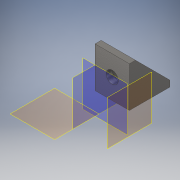
# Autodesk Inventor part: Corner Piece
Saved by Autodesk Inventor 2017 (Build 210142000, 142)
## iProperties
Part Number: Corner Piece
Material: Aluminum 6061-AHC
Document SubType Name: Modeling
Designer: Till
Density: 2.7 g/cm^3
Appearance: Galvanisiert
Author: Till
Autodesk Inventor part; units mm, degrees
ref_plane "YZ Plane" through (0, 0, 0) normal (1, 0, 0) x (0, 1, 0)
ref_plane "XZ Plane" through (0, 0, 0) normal (0, 1, 0) x (-1, 0, 0)
ref_plane "XY Plane" through (0, 0, 0) normal (0, 0, 1) x (1, 0, 0)
ref_plane "Arbeitsebene7" through (0, 0, 0) normal (0, 0, 1) x (1, 0, 0)
sketch "Skizze1" plane through (0, 0, 0) normal (0, 0, 1) x (1, 0, 0)
  line L0 (12, 20) -> (17, 20) projected
  line L1 (0, 20) -> (5, 20) projected
  line L2 (17, 20) -> (0, 20)
  line L3 (0, 20) -> (0, 40)
  line L4 (0, 40) -> (17, 40)
  line L5 (17, 40) -> (17, 20)
  point P0 (0, 0)
  dimension "d0" = 20
  constraints: 8 end point, 3 perpendicular, 1 collinear
  measures "d0" distance of L1.start L3.end
extrude "Extrusion1" add sketch "Skizze1" along normal blind 3
ref_plane "Arbeitsebene6" through (5, 20, 0) normal (0, 1, 0) x (-1, 0, 0)
sketch "Skizze2" plane through (5, 20, 0) normal (0, 1, 0) x (-1, 0, 0)
  line L0 (-12, 0) -> (-12, 400) projected
  line L1 (5, 3) -> (-12, 3) projected
  line L2 (-12, 3) -> (5, 3)
  line L3 (5, 3) -> (5, 20)
  line L4 (5, 20) -> (-12, 20)
  line L5 (-12, 20) -> (-12, 3)
  point P0 (5, 0)
  dimension "d3" = 17
  constraints: 8 end point, 2 parallel, 1 horizontal, 1 perpendicular
  measures "d3" distance of L3.end L2.end
extrude "Extrusion2" add sketch "Skizze2" along normal blind 3
ref_plane "Arbeitsebene5" through (0, 20, 0) normal (-1, 0, 0) x (0, 0, 1)
sketch "Skizze4" plane through (0, 20, 0) normal (-1, 0, 0) x (0, 0, 1)
  line L0 (3, 3) -> (3, 20) projected
  line L1 (20, 3) -> (3, 3) projected
  line L2 (3, 20) -> (20, 3)
  line L3 (20, 3) -> (3, 3)
  line L4 (0, 20) -> (3, 20) projected
  line L5 (3, 3) -> (3, 20)
  point P0 (0, -20)
  constraints: 6 end point, 1 collinear, 1 perpendicular
extrude "Extrusion3" add sketch "Skizze4" against normal blind 3
ref_plane "Arbeitsebene4" through (17, 20, 0) normal (1, 0, 0) x (0, 0, -1)
sketch "Skizze5" plane through (17, 20, 0) normal (1, 0, 0) x (0, 0, -1)
  line L0 (-3, 3) -> (-3, 20) projected
  line L1 (-3, 20) -> (-3, 3)
  line L2 (-20, 3) -> (-3, 3) projected
  line L3 (-3, 3) -> (-20, 3)
  line L4 (-3, 20) -> (-20, 3) projected
  line L5 (-20, 3) -> (-3, 20)
  point P0 (0, -20)
  constraints: 6 end point, 3 collinear
extrude "Extrusion4" add sketch "Skizze5" against normal blind 3
hole "Bohrung3" at (8.5, 30, 3) direction (0, 0, -1) diameter 6 end through all
hole "Bohrung4" at (8.5, 23, 10) direction (0, -1, 0) diameter 6 end through all
